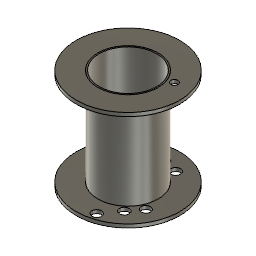
birdcage_rat_head (Autodesk Fusion 360 design; units mm, degrees)
Autodesk Fusion 360 part; units mm, degrees
sketch "Sketch1" plane through (0, 0, 0) normal (0, 0, 1) x (1, 0, 0)
  circle A0 centre (0, 0) radius 21
  circle A1 centre (0, 0) radius 20
  circle A2 centre (0, 0) radius 36.25
  circle A3 centre (0, 0) radius 36.5
  circle A4 centre (0, 0) radius 37.5
  circle A5 centre (16.5555, -19.0651) radius 3.325
  circle A6 centre (10.477, 22.9738) radius 3.325
  circle A7 centre (23.6561, 8.8291) radius 2.5
  circle A8 centre (8.3264, -30.1618) radius 3.325
  circle A9 centre (-13.5897, 28.1848) radius 3.25
  circle A10 centre (22.9738, -10.477) radius 3.25
  circle A11 centre (0, 25.25) radius 3.325
  dimension "d1" = 42
  dimension "d6" = 72.5
  dimension "d10" = 40
  dimension "d68" = 73
  dimension "d69" = 75
  dimension "d77" = 6.65
  dimension "d78" = 6.65
  dimension "d80" = 5
  dimension "d81" = 6.65
  dimension "d82" = 6.5
  dimension "d83" = 6.5
  dimension "d84" = 6.65
  constraint coincident A0.centre A1.centre
  constraint concentric A0 A1
  constraint concentric A0 A2
  constraint concentric A2 A3
  measures "d1" diameter of A0
  measures "d6" diameter of A2
  measures "d10" diameter of A1
  measures "d68" diameter of A3
  measures "d69" diameter of A4
  measures "d77" diameter of A5
  measures "d78" diameter of A6
  measures "d80" diameter of A7
  measures "d81" diameter of A8
  measures "d82" diameter of A9
  measures "d83" diameter of A10
  measures "d84" diameter of A11
extrude "Extrude2" add sketch "Sketch1" along normal blind 70 contours A0 makes body 1
extrude "Extrude4" add sketch "Sketch1" against normal blind 2.5 separate body contours A2 | A5 | A6 | A7 | A8 | A9 | A10 | A11 makes body 2
hole "Hole10" [suppressed]
copy_body "CopyPasteBodies1" bodies 2 makes body 3
move_body "Move1" bodies 3 to x (1, 0, 0) y (0, 1, 0) z (0, 0, 1) at (0, 0, 43.5)
move_body "Move2" bodies 1 to x (1, 0, 0) y (0, 1, 0) z (0, 0, 1) at (0, 0, -3.5)
extrude "Extrude6" add sketch "Sketch1" along normal blind 64 separate body contours A4 makes body 4
move_body "Move3" bodies 4 to x (1, 0, 0) y (0, 1, 0) z (0, 0, 1) at (0, 0, -3.5)
draft "Draft1" angle -0.6 neutral plane through (0, 0, 0) pull (0, 0, 1) 1 faces at (-36.3186, -3.6342, 17.8333) on bodies 4
move_body "Move4" bodies 2 to x (1, 0, 0) y (0, 1, 0) z (0, 0, 1) at (0, 0, -0.9)
move_body "Move6" bodies 3 to x (1, 0, 0) y (0, 1, 0) z (0, 0, 1) at (0, 0, 18.59)
move_body "Align1" bodies 3 to x (1, 0, 0) y (0, 1, 0) z (0, 0, 1) at (0, 0, 4.41)
extrude "Extrude8" add sketch "Sketch1" along normal blind 2.6 separate body contours A9 makes body 5
extrude "Extrude9" add sketch "Sketch1" along normal blind 2.6 separate body contours A8 makes body 6
extrude "Extrude10" add sketch "Sketch1" along normal blind 2.6 separate body contours A5 makes body 7
extrude "Extrude11" add sketch "Sketch1" along normal blind 2.6 separate body contours A10 makes body 8
extrude "Extrude14" add sketch "Sketch1" along normal blind 2.6 separate body contours A11 makes body 9
move_body "Align2" bodies 5 to x (1, 0, 0) y (0, 1, 0) z (0, 0, 1) at (0, 0, -3.4)
combine "Combine1" operation cut target body 2 tool bodies 5 keep tools
move_body "Align3" bodies 9 to x (1, 0, 0) y (0, 1, 0) z (0, 0, 1) at (0, 0, -3.4)
combine "Combine2" operation cut target body 2 tool bodies 9 keep tools
extrude "Extrude15" add sketch "Sketch1" against normal blind 2.6 separate body contours A6 makes body 10
move_body "Align5" bodies 10 to x (1, 0, 0) y (0, 1, 0) z (0, 0, 1) at (0, 0, -0.9)
combine "Combine3" operation cut target body 2 tool bodies 10 keep tools
move_body "Align6" bodies 6 to x (1, 0, 0) y (0, 1, 0) z (0, 0, 1) at (0, 0, -3.5)
combine "Combine4" operation cut target body 2 tool bodies 6 keep tools
move_body "Align7" bodies 8 to x (1, 0, 0) y (0, 1, 0) z (0, 0, 1) at (0, 0, -3.5)
combine "Combine5" operation cut target body 2 tool bodies 8 keep tools
move_body "Align8" bodies 7 to x (1, 0, 0) y (0, 1, 0) z (0, 0, 1) at (0, 0, -3.5)
combine "Combine6" operation cut target body 2 tool bodies 7 keep tools
extrude "Extrude16" add sketch "Sketch1" along normal blind 2.6 separate body contours A7 makes body 11
move_body "Align9" bodies 11 to x (1, 0, 0) y (0, 1, 0) z (0, 0, 1) at (0, 0, 63.9)
combine "Combine7" operation cut target body 3 tool bodies 11 keep tools
move_body "Align10" bodies 2 to x (1, 0, 0) y (0, 1, 0) z (0, 0, 1) at (0, 0, -0.1)
moveface "MoveFace1" [suppressed]
extrude "Extrude5" [suppressed]
hole "Hole3" [suppressed]
hole "Hole4" [suppressed]
hole "Hole5" [suppressed]
hole "Hole6" [suppressed]
hole "Hole7" [suppressed]
hole "Hole8" [suppressed]
hole "Hole9" [suppressed]
hole "Hole2" [suppressed]
hole "Hole1" [suppressed]
extrude "Extrude1" [suppressed]
sketch "Sketch2" plane through (0, 0, 0) normal (0, 0, 1) x (1, 0, 0)
hidden bodies 4 5 6 7 8 9 10 11
equation "d1 = 27 mm + 15 mm"
equation "d6 = 57.5 mm + 15 mm"
equation "d10 = 25 mm + 15 mm"
equation "d68 = 58 mm + 15 mm"
equation "d69 = 60 mm + 15 mm"
named bodies: "central cylinder", "rf_flange", "balance flange", "inner shell", "0- jack", "90 tune", "90 match", "90 jack", "0 match", "0 tune"
